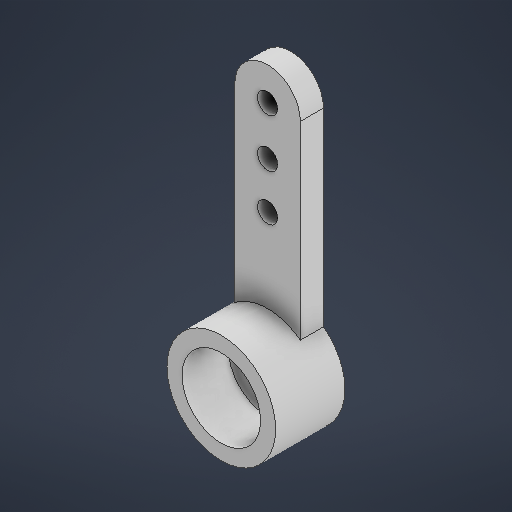
# Autodesk Inventor part: 摆臂
Saved by Autodesk Inventor 2025 (Build 290162000, 162)
## iProperties
Created: 2025-12-07
Part Number: 摆臂
Material: 常规
Document SubType Name: Modeling
Designer: XH
Density: 1 g/cm^3
Appearance: 默认
Author: XH
Autodesk Inventor part; units mm, degrees
ref_plane "YZ Plane" through (0, 0, 0) normal (1, 0, 0) x (0, 1, 0)
ref_plane "XZ Plane" through (0, 0, 0) normal (0, 1, 0) x (-1, 0, 0)
ref_plane "XY Plane" through (0, 0, 0) normal (0, 0, 1) x (1, 0, 0)
sketch "草图1" plane through (0, 0, 0) normal (0, 0, 1) x (1, 0, 0)
  circle A0 centre (0, 0) radius 2.7
  circle A1 centre (0, 0) radius 1.6
  line L0 (0, 0) -> (0, 11.5707) construction
  line L1 (1.6293, 0) -> (1.6293, 11.5707)
  line L2 (-1.6293, 11.5707) -> (-1.6293, 0)
  arc A2 (-1.6293, 0) -> (1.6293, 0) centre (0, 0) ccw
  arc A3 (1.6293, 11.5707) -> (-1.6293, 11.5707) centre (0, 11.5707) ccw
  point P0 (0, 5.7853)
  point P1 (0, 13.2)
  point P2 (0, -2.7)
  point P3 (-1.6293, 2.153)
  point P4 (1.6293, 2.153)
  dimension "d0" = 5.4
  dimension "d1" = 3.2
  dimension "d2" = 15.9
  constraints: 8 end point, 5 point on circle, 4 tangent, 3 centre point, 2 coincident, 1 midpoint, 1 parallel, 1 vertical, 3 other
  measures "d1" diameter of A1
  measures "d2" distance of point (0, 13.2) point (0, -2.7)
extrude "拉伸1" add sketch "草图1" along normal blind 1.15 contours A0 L2 A2 L1 | L1 A2 L2 A0 | A0 L2 A3 L1 | A1
sketch "草图2" plane through (0, 0, 1.15) normal (0, 0, 1) x (1, 0, 0)
  circle A0 centre (0, 0) radius 1.95
  circle A1 centre (0, 0) radius 2.7
  dimension "d5" = 3.9
  constraints: 2 centre point, 2 coincident
  measures "d5" diameter of A0
extrude "拉伸2" add sketch "草图2" along normal blind 2.3
sketch "草图3" plane through (0, 0, 1.15) normal (0, 0, 1) x (1, 0, 0)
  circle A0 centre (0, 11.5462) radius 0.5
  circle A1 centre (0, 9.1462) radius 0.5
  circle A2 centre (0, 6.85) radius 0.5
  circle A3 centre (0, 0) radius 1.95 projected
  dimension "d8" = 1
  dimension "d9" = 1
  dimension "d10" = 1
  dimension "d12" = 6.85
  dimension "d13" = 2.4
  constraints: 3 centre point
  measures "d8" diameter of A0
  measures "d9" diameter of A1
  measures "d10" diameter of A2
  measures "d12" distance of A2.centre A3.centre
  measures "d13" distance of A0.centre A1.centre
extrude "拉伸3" cut sketch "草图3" against normal blind 2.3 contours A0 | A1 | A2
